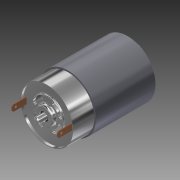
# Autodesk Inventor part: RS-775
Saved by Autodesk Inventor 2013 (Build 170138000, 138)
## iProperties
Category: Motors
Company: Autodesk, Inc.
Shininess: 64.0
Length Units: 11272
Angle Units: 11279
Time Units: 11290
Mass Units: 11286
Length Display Precision: 3
Angle Display Precision: 2
Compacted: True
Part Number: RS-775
Document SubType Name: Modeling
Created: 2011-12-15
Material: Steel, Mild
Project: FIRST
Catalog Web Link: http://banebots.com/pc/FIRST/M7-RS775-18
Vendor: BaneBots
Density: 13.8052 g/cm^3
Description: Motor - BaneBots RS-775
Mass: 337 g
Surface Area: 246.039 cm^2
Volume: 24.4112 cm^3
Density: 0.0
Volumn: 0.0
Area: 0.0
PropertySet Name: Model Information
Control State: 0
Master: False
Checked Out: False
Title: Motor - BaneBots RS-775
Author: Autodesk, Inc.
Autodesk Inventor part; units mm, degrees
sketch "Sketch1" plane through (0, 0, 0) normal (0, 0, 1) x (1, 0, 0)
  circle A0 centre (0, 0) radius 21.05
  dimension "d0" = 42.1
  constraints: 2 coincident, 1 centre point, 2 other
  measures "d0" diameter of A0
extrude "Extrusion1" add sketch "Sketch1" along normal mid plane 66.548
fillet "Fillet1" radius 2 1 edges at (-21.05, 0, 33.274)
shell "Shell1" thickness 0.62 removed faces 1 at (3.9859, -5.7746, -33.274)
sketch "Sketch2" plane through (0, 0, 33.274) normal (0, 0, 1) x (1, 0, 0)
  circle A0 centre (0, 0) radius 19.05 projected
  circle A1 centre (0, 0) radius 6.5
  dimension "d5" = 13
  constraints: 1 centre point, 1 coincident, 1 concentric
  measures "d5" diameter of A1
extrude "Extrusion2" add sketch "Sketch2" along normal blind 4.5 contours A1
fillet "Fillet2" radius 0.5 2 edges at (-6.5, 0, 33.274) (-6.5, 0, 37.774)
sketch "Sketch3" plane through (0, 0, 37.774) normal (0, 0, 1) x (1, 0, 0)
  circle A0 centre (0, 0) radius 6 projected
  circle A1 centre (0, 0) radius 2.5
  dimension "d9" = 5
  constraints: 1 centre point, 1 coincident, 1 concentric
  measures "d9" diameter of A1
extrude "Extrusion3" add sketch "Sketch3" along normal blind 7.6 contours A1
fillet "Fillet3" radius 2.5 1 edges at (-2.5, 0, 45.374)
sketch "Sketch4" plane through (0, 0, 33.274) normal (0, 0, 1) x (1, 0, 0)
  circle A0 centre (0, 0) radius 19.05 projected
  point P0 (12.5, 0)
  dimension "d13" = 12.5
  constraints: 1 horizontal alignment
  measures "d13" distance of point (12.5, 0) A0.centre
hole "Hole1" at (12.5, 0, 33.274) direction (0, 0, -1) diameter 2.5 depth 8 tip angle 118
mirror "Mirror1" about plane through (0, 0, 0) normal (1, 0, 0) of "Hole1"
sketch "Sketch5" plane through (0, 0, 33.274) normal (0, 0, 1) x (1, 0, 0)
  circle A0 centre (12.5, 0) radius 1.25 projected
  circle A1 centre (0, 0) radius 7 projected
  arc A2 (15.4548, 4.1411) -> (4.1411, 15.4548) centre (0, 0) ccw
  arc A3 (11.5911, 3.1058) -> (3.1058, 11.5911) centre (0, 0) ccw
  line L0 (0, 0) -> (4.1411, 15.4548) construction
  line L1 (0, 0) -> (15.4548, 4.1411) construction
  line L2 (3.1058, 11.5911) -> (4.1411, 15.4548)
  line L3 (11.5911, 3.1058) -> (15.4548, 4.1411)
  line L4 (0, 0) -> (12.5, 0) construction
  line L5 (0.151, 0.5634) -> (0.151, 14.7153) construction
  dimension "d21" = 15
  dimension "d22" = 15
  dimension "d23" = 16
  dimension "d24" = 12
  constraints: 12 end point, 4 point on circle, 3 point on line, 2 centre point, 2 coincident, 2 collinear, 2 concentric, 1 horizontal, 1 perpendicular
  measures "d21" angle of L1 L4
  measures "d22" angle of L5 L0
  measures "d23" radius of A2
  measures "d24" radius of A3
extrude "Extrusion4" cut sketch "Sketch5" against normal blind 10 contours L3 A3 L2 A2
pattern_circular "Circular Pattern1" count 4 over 360 about axis through (0, 0, 0) along (0, 0, 1) of "Extrusion4"
ref_plane "Work Plane1" through (0, 0, -31.369) normal (0, 0, -1) x (-1, 0, 0)
sketch "Sketch6" plane through (0, 0, -31.369) normal (0, 0, -1) x (-1, 0, 0)
  circle A0 centre (0, 0) radius 20.43 projected
extrude "Extrusion5" add sketch "Sketch6" against normal blind 0.62
sketch "Sketch7" plane through (0, 0, -31.369) normal (0, 0, -1) x (-1, 0, 0)
  circle A0 centre (0, 0) radius 20.43 projected
  circle A1 centre (0, 0) radius 12.7
  dimension "d33" = 25.4
  constraints: 1 centre point, 1 coincident, 1 concentric
  measures "d33" diameter of A1
extrude "Extrusion6" add sketch "Sketch7" along normal blind 1.27 draft -2.5 contours A1
fillet "Fillet4" radius 0.508 1 edges at (12.7, 0, -31.369)
fillet "Fillet5" radius 0.508 1 edges at (12.6446, 0, -32.639)
sketch "Sketch16" plane through (0, 0, -32.639) normal (0, 0, -1) x (-1, 0, 0)
  circle A0 centre (0, 0) radius 12.4207
  arc A1 (10.4533, 1.8432) -> (11.5431, 3.639) centre (10.2107, 3.219) ccw
  line L0 (10.4155, 1.8365) -> (10.4533, 1.8432)
  arc A2 (8.8407, 2.7916) -> (10.4155, 1.8365) centre (10.1729, 3.2123) ccw
  arc A3 (8.8407, 2.7916) -> (4.2844, 8.2216) centre (0, 0) ccw
  arc A4 (3.6173, 9.9383) -> (4.2844, 8.2216) centre (4.93, 9.4605) ccw
  line L1 (3.6304, 9.9744) -> (3.6173, 9.9383)
  arc A5 (5.5882, 10.7358) -> (3.6304, 9.9744) centre (4.9431, 9.4966) ccw
  arc A6 (11.5431, 3.639) -> (5.5882, 10.7358) centre (0, 0) ccw
  arc A7 (3.6304, -9.9744) -> (5.5882, -10.7358) centre (4.9431, -9.4966) ccw
  line L2 (3.6173, -9.9383) -> (3.6304, -9.9744)
  arc A8 (4.2844, -8.2216) -> (3.6173, -9.9383) centre (4.93, -9.4605) ccw
  arc A9 (4.2844, -8.2216) -> (8.8407, -2.7916) centre (0, 0) ccw
  arc A10 (10.4155, -1.8365) -> (8.8407, -2.7916) centre (10.1729, -3.2123) ccw
  line L3 (10.4533, -1.8432) -> (10.4155, -1.8365)
  arc A11 (11.5431, -3.639) -> (10.4533, -1.8432) centre (10.2107, -3.219) ccw
  arc A12 (5.5882, -10.7358) -> (11.5431, -3.639) centre (0, 0) ccw
  circle A13 centre (0, 0) radius 8.2169
  line L4 (-3.6173, -9.9383) -> (-3.6304, -9.9744)
  arc A14 (-5.5882, -10.7358) -> (-3.6304, -9.9744) centre (-4.9431, -9.4966) ccw
  arc A15 (-11.5431, -3.639) -> (-5.5882, -10.7358) centre (0, 0) ccw
  arc A16 (-10.4533, -1.8432) -> (-11.5431, -3.639) centre (-10.2107, -3.219) ccw
  line L5 (-10.4533, -1.8432) -> (-10.4155, -1.8365)
  arc A17 (-8.8407, -2.7916) -> (-10.4155, -1.8365) centre (-10.1729, -3.2123) ccw
  arc A18 (-8.8407, -2.7916) -> (-4.2844, -8.2216) centre (0, 0) ccw
  arc A19 (-3.6173, -9.9383) -> (-4.2844, -8.2216) centre (-4.93, -9.4605) ccw
  line L6 (-10.4155, 1.8365) -> (-10.4533, 1.8432)
  arc A20 (-11.5431, 3.639) -> (-10.4533, 1.8432) centre (-10.2107, 3.219) ccw
  arc A21 (-5.5882, 10.7358) -> (-11.5431, 3.639) centre (0, 0) ccw
  arc A22 (-3.6304, 9.9744) -> (-5.5882, 10.7358) centre (-4.9431, 9.4966) ccw
  line L7 (-3.6304, 9.9744) -> (-3.6173, 9.9383)
  arc A23 (-4.2844, 8.2216) -> (-3.6173, 9.9383) centre (-4.93, 9.4605) ccw
  arc A24 (-4.2844, 8.2216) -> (-8.8407, 2.7916) centre (0, 0) ccw
  arc A25 (-10.4155, 1.8365) -> (-8.8407, 2.7916) centre (-10.1729, 3.2123) ccw
  circle A26 centre (0, 0) radius 3.2359
  constraints: 48 point on circle, 27 centre point, 16 end point
extrude "Extrusion14" cut sketch "Sketch16" against normal up to next contours L0 A2 A3 A4 L1 A5 A6 A1 | L2 A8 A9 A10 L3 A11 A12 A7 | L4 A14 A15 A16 L5 A17 A18 A19 | L6 A20 A21 A22 L7 A23 A24 A25
sketch "Sketch8" plane through (0, 0, -32.639) normal (0, 0, -1) x (-1, 0, 0)
  circle A0 centre (0, 0) radius 12.6446 projected
  circle A1 centre (0, 0) radius 7.4549
  dimension "d36" = 14.9098
  constraints: 1 centre point, 1 coincident, 1 concentric
  measures "d36" diameter of A1
extrude "Extrusion7" add sketch "Sketch8" along normal blind 3 contours A1
sketch "Sketch9" plane through (0, 0, -35.639) normal (0, 0, -1) x (-1, 0, 0)
  circle A0 centre (0, 0) radius 7.4549 projected
  circle A1 centre (0, 0) radius 3.45
  dimension "d39" = 6.9
  constraints: 1 centre point, 1 coincident, 1 concentric
  measures "d39" diameter of A1
extrude "Extrusion8" cut sketch "Sketch9" against normal blind 0.8 contours A1
sketch "Sketch10" plane through (0, 0, -34.839) normal (0, 0, -1) x (-1, 0, 0)
  circle A0 centre (0, 0) radius 3.45 projected
  circle A1 centre (0, 0) radius 2.4638
  dimension "d42" = 4.9276
  constraints: 1 centre point, 1 coincident, 1 concentric
  measures "d42" diameter of A1
extrude "Extrusion9" add sketch "Sketch10" along normal blind 7.4422 contours A1
sketch "Sketch12" plane through (0, 0, -31.369) normal (0, 0, -1) x (-1, 0, 0)
  circle A0 centre (0, 0) radius 12.7 projected
  circle A1 centre (0, 0) radius 20.43 projected
  line L0 (-18.4197, 2.4638) -> (-17.9197, 2.4638)
  line L1 (-17.9197, 2.4638) -> (-17.9197, -2.4638)
  line L2 (-17.9197, -2.4638) -> (-18.4197, -2.4638)
  line L3 (-18.4197, -2.4638) -> (-18.4197, 2.4638)
  line L4 (0, 0) -> (-16.9017, 0) construction
  point P0 (-17.9197, 0)
  dimension "d54" = 0.5
  dimension "d55" = 4.9276
  dimension "d56" = 17.9197
  constraints: 10 end point, 2 parallel, 2 perpendicular, 1 horizontal, 1 midpoint, 1 point on line
  measures "d54" distance of L1.end L2.end
  measures "d55" distance of L2.end L0.start
  measures "d56" distance from line of L1 A0.centre
extrude "Extrusion11" add sketch "Sketch12" along normal blind 11.43 contours L0 L1 L2 L3
chamfer "Chamfer1" distance 1 angle 45 2 edges at (18.1697, 2.4638, -42.799) (18.1697, -2.4638, -42.799)
sketch "Sketch13" plane through (18.4197, -2.4638, -31.369) normal (1, 0, 0) x (0, 0, -1)
  line L0 (11.43, 1) -> (11.43, 3.9276) projected
  line L1 (8.43, 2.4638) -> (10.43, 4.9276) construction
  line L2 (8.43, 2.4638) -> (10.43, 0) construction
  dimension "d61" = 3
  constraints: 4 end point, 1 equal length
  measures "d61" distance from line of L0 L1.start
hole "Hole2" at (18.4197, 0, -39.799) direction (-1, 0, 0) diameter 2 depth 1 tip angle 118
mirror "Mirror2" about plane through (0, 0, 0) normal (1, 0, 0) of "Extrusion11", "Chamfer1", "Hole2"
ref_plane "Work Plane2" through (18, 0, 0) normal (1, 0, 0) x (0, 1, 0)
ref_plane "Work Plane3" through (0, 0, 31.274) normal (0, 0, -1) x (-1, 0, 0)
sketch "Sketch15" plane through (0, 0, 31.274) normal (0, 0, -1) x (-1, 0, 0)
  circle A0 centre (0, 0) radius 21.05 projected
  circle A1 centre (0, 0) radius 22.2565
  dimension "d76" = 1.2065
  constraints: 1 centre point
  measures "d76" radial gap between concentric circles of A1 A0
extrude "Flux Ring" add sketch "Sketch15" along normal blind 47.5
fillet "Fillet6" radius 0.762 1 edges at (7.4549, 0, -32.639)
fillet "Fillet7" radius 1.27 1 edges at (7.4549, 0, -35.639)
fillet "Fillet8" radius 1.27 1 edges at (2.4638, 0, -42.2812)
body "Solid1"
